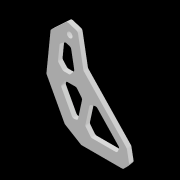
# Autodesk Inventor part: upper-arm-bracket
Saved by Autodesk Inventor 2020 (Build 240168000, 168)
## iProperties
Created: 2020-03-28
Part Number: upper-arm-bracket
Material: Generic
Document SubType Name: Modeling
Designer: valer
Density: 1 g/cm^3
Appearance: Default
Author: valer
Autodesk Inventor part; units mm, degrees
ref_plane "YZ Plane" through (0, 0, 0) normal (1, 0, 0) x (0, 1, 0)
ref_plane "XZ Plane" through (0, 0, 0) normal (0, 1, 0) x (-1, 0, 0)
ref_plane "XY Plane" through (0, 0, 0) normal (0, 0, 1) x (1, 0, 0)
sketch "Base" plane through (0, 0, 0) normal (0, 0, 1) x (1, 0, 0)
  line L0 (-68.58, 0) -> (0, 0)
  line L1 (0, 0) -> (-4.3619, 22.44)
  line L2 (-4.3619, 22.44) -> (-53.3177, 74.0286)
  line L3 (-95.2508, 50.1605) -> (-68.58, 0)
  line L4 (-95.2508, 50.1605) -> (-90.4866, 95.4894)
  line L5 (-59.798, 108.9932) -> (-71.9102, 112.8121)
  line L6 (-71.9102, 112.8121) -> (-90.4866, 95.4894)
  line L7 (-59.798, 108.9932) -> (-53.3177, 74.0286)
  line L8 (-38.7127, 46.3383) -> (-12.6192, 18.8415)
  line L9 (-46.3383, 44.2062) -> (-51.3858, 20.9737)
  line L10 (-44.7167, 12.7) -> (-15.2578, 12.7)
  line L11 (-46.3383, 44.2062) -> (-38.7127, 46.3383)
  line L12 (-15.2578, 12.7) -> (-12.6192, 18.8415)
  line L13 (-44.7167, 12.7) -> (-51.3858, 20.9737)
  line L14 (-74.3842, 53.8912) -> (-61.365, 53.8912)
  line L15 (-54.6958, 45.6176) -> (-59.7894, 22.1732)
  line L16 (-78.876, 46.4156) -> (-65.5618, 21.3752)
  line L17 (-65.5618, 21.3752) -> (-59.7894, 22.1732)
  line L18 (-61.365, 53.8912) -> (-54.6958, 45.6176)
  line L19 (-78.876, 46.4156) -> (-74.3842, 53.8912)
  line L20 (-80.2456, 87.3078) -> (-82.2041, 68.6731)
  line L21 (-67.4696, 89.8041) -> (-63.5399, 68.6015)
  line L22 (-76.5179, 62.3579) -> (-68.7327, 62.3579)
  line L23 (-73.5257, 91.7136) -> (-67.4696, 89.8041)
  line L24 (-82.2041, 68.6731) -> (-76.5179, 62.3579)
  line L25 (-68.7327, 62.3579) -> (-63.5399, 68.6015)
  line L26 (-80.2456, 87.3078) -> (-73.5257, 91.7136)
  line L27 (0, -22.5624) -> (0, 135.3746) construction
  line L28 (-114.301, 0) -> (19.0502, 0) construction
  point P0 (-74.2784, 89.0258)
  point P1 (-44.5408, 52.4798)
  point P2 (-6.7911, 12.7)
  point P3 (-53.1833, 12.7)
  point P4 (-82.8508, 53.8912)
  point P5 (-52.8983, 53.8912)
  point P6 (-61.5869, 13.8996)
  point P7 (-52.8983, 53.8912)
  point P8 (-79.5818, 93.623)
  point P9 (-82.8679, 62.3579)
  point P10 (-62.3827, 62.3579)
  dimension "d0" = 8.4667
  dimension "d1" = 8.4667
  dimension "d2" = 8.4667
  dimension "d3" = 8.4667
  dimension "d4" = 8.4667
  dimension "d5" = 8.4667
  dimension "d6" = 8.4667
  dimension "d7" = 8.4667
  dimension "d8" = 8.4667
  dimension "d9" = 8.4667
  dimension "d10" = 8.4667
  dimension "d11" = 8.4667
  dimension "d12" = 6.35
  dimension "d13" = 6.35
  dimension "d14" = 6.35
  dimension "d15" = 6.35
  dimension "d16" = 6.35
  dimension "d17" = 6.35
  dimension "d18" = 11
  dimension "d19" = 43.5
  dimension "d20" = 147
  dimension "d21" = 118
  dimension "d22" = 119.5
  dimension "d23" = 139
  dimension "d24" = 62
  dimension "d25" = 68.58
  dimension "d26" = 22.86
  dimension "d27" = 8.4667
  dimension "d28" = 8.4667
  dimension "d29" = 71.12
  dimension "d30" = 35.56
  dimension "d31" = 12.7
  dimension "d32" = 25.4
  dimension "d33" = 12.7
  dimension "d34" = 12.7
  dimension "d35" = 11.0401
  dimension "d36" = 11.0401
  dimension "d37" = 6.35
  dimension "d38" = 7.7852
  dimension "d39" = 8.4667
  constraints: 54 end point, 20 point on line, 6 parallel, 5 horizontal, 1 other
  measures "d0" distance of L9.start point (-44.541, 52.48)
  measures "d1" distance of L11.end point (-44.541, 52.48)
  measures "d2" distance of L10.end point (-6.791, 12.7)
  measures "d3" distance of L8.end point (-6.791, 12.7)
  measures "d4" distance of L13.start point (-53.183, 12.7)
  measures "d5" distance of L9.end point (-53.183, 12.7)
  measures "d6" distance of L17.start point (-61.587, 13.9)
  measures "d7" distance of L15.end point (-61.587, 13.9)
  measures "d8" distance of L18.start point (-52.898, 53.891)
  measures "d9" distance of L15.start point (-52.898, 53.891)
  measures "d10" distance of L19.start point (-82.851, 53.891)
  measures "d11" distance of L14.start point (-82.851, 53.891)
  measures "d12" distance of L20.end point (-82.868, 62.358)
  measures "d13" distance of L24.end point (-82.868, 62.358)
  measures "d14" distance of L22.end point (-62.383, 62.358)
  measures "d15" distance of L21.end point (-62.383, 62.358)
  measures "d16" distance of L26.start point (-79.582, 93.623)
  measures "d17" distance of L23.start point (-79.582, 93.623)
  measures "d18" angle of L27 L1
  measures "d19" angle of L27 L2
  measures "d20" angle of L2 L7
  measures "d21" angle of L7 L5
  measures "d22" angle of L5 L6
  measures "d23" angle of L4 L6
  measures "d24" angle of L28 L3
  measures "d25" distance of L0.start L0.end
  measures "d26" distance of L0.end L1.end
  measures "d27" distance between parallel lines of L2 L8
  measures "d28" distance between parallel lines of L15 L9
  measures "d29" distance of L1.end L2.end
  measures "d30" distance of L5.start L2.end
  measures "d31" distance of L5.start L5.end
  measures "d32" distance of L5.end L6.end
  measures "d33" distance between parallel lines of L0 L10
  measures "d34" distance between parallel lines of L3 L16
  measures "d35" distance between parallel lines of L7 L21
  measures "d36" distance between parallel lines of L4 L20
  measures "d37" distance of L23.start L23.end
  measures "d38" distance of L24.end L22.end
  measures "d39" distance between parallel lines of L14 L22
extrude "Extrusion1" add sketch "Base" along normal mid plane 5.08
chamfer "Chamfer1" distance 8.4667 angle 45 1 edges at (0, 0, 0)
sketch "Sketch2" plane through (0, 0, 2.54) normal (0, 0, 1) x (1, 0, 0)
  circle A0 centre (-68.9092, 101.2129) radius 3.175
  line L0 (-59.798, 108.9932) -> (-71.9102, 112.8121) construction
  line L1 (-71.9102, 112.8121) -> (-59.798, 108.9932) projected
  line L2 (-65.8541, 110.9026) -> (-68.9092, 101.2129) construction
  point P0 (0, 0)
  dimension "d45" = 6.35
  dimension "d46" = 10.16
  constraints: 2 end point, 1 centre point, 1 coincident, 1 midpoint, 1 perpendicular
  measures "d45" diameter of A0
  measures "d46" distance of L2.start L2.end
hole "UpperArmMountHoleFeature" at (-68.9092, 101.2129, 2.54) direction (0, 0, -1) diameter 6.35 end through all
chamfer "Chamfer2" distance 12.7 angle 45 1 edges at (-68.58, 0, 0)
fillet "Fillet1" radius 2.54 29 edges at (-59.7894, 22.1732, 0) (-54.6958, 45.6176, 0) (-61.365, 53.8912, 0) (-74.3842, 53.8912, 0) (-78.876, 46.4156, 0) (-65.5618, 21.3752, 0) (-76.5179, 62.3579, 0) (-82.2041, 68.6731, 0) (-80.2456, 87.3078, 0) (-68.7327, 62.3579, 0) (-63.5399, 68.6015, 0) (-67.4696, 89.8041, 0) (-73.5257, 91.7136, 0) (-15.2578, 12.7, 0) (-12.6192, 18.8415, 0) (-38.7127, 46.3383, 0) (-46.3383, 44.2062, 0) (-51.3858, 20.9737, 0) (-44.7167, 12.7, 0) (-4.3619, 22.44, 0) (-1.6155, 8.3111, 0) (-8.4667, 0, 0) (-55.88, 0, 0) (-74.5423, 11.2134, 0) (-95.2508, 50.1605, 0) (-90.4866, 95.4894, 0) (-71.9102, 112.8121, 0) (-59.798, 108.9932, 0) (-53.3177, 74.0286, 0)
equation "\"d1\" = d0"
equation "\"d3\" = d2"
equation "\"d4\" = d2"
equation "\"d5\" = d4"
equation "\"d7\" = d6"
equation "\"d8\" = d6"
equation "\"d9\" = d8"
equation "\"d10\" = d6"
equation "\"d11\" = d10"
equation "\"d13\" = d12"
equation "\"d14\" = d12"
equation "\"d15\" = d14"
equation "\"d16\" = d12"
equation "\"d17\" = d16"
equation "\"d36\" = d35"
body "Solid1"
